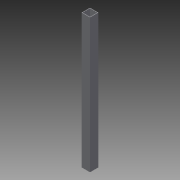
# Autodesk Inventor part: Part15-01
Saved by Autodesk Inventor 2013 (Build 170138000, 138)
## iProperties
Created: 2012-10-21
Part Number: Part15-01
Material: Generic
Document SubType Name: Modeling
Designer: Istvan
Density: 1 g/cm^3
Author: Istvan
Autodesk Inventor part; units mm, degrees
ref_plane "YZ Plane" through (0, 0, 0) normal (1, 0, 0) x (0, 1, 0)
ref_plane "XZ Plane" through (0, 0, 0) normal (0, 1, 0) x (-1, 0, 0)
ref_plane "XY Plane" through (0, 0, 0) normal (0, 0, 1) x (1, 0, 0)
sketch "Sketch1" plane through (0, 0, 0) normal (0, 1, 0) x (-1, 0, 0)
  line L0 (0, 0) -> (-38.1, 0)
  line L1 (-38.1, 0) -> (-38.1, -38.1)
  line L2 (-38.1, -38.1) -> (0, -38.1)
  line L3 (0, -38.1) -> (0, 0)
  line L4 (-35.7188, -35.7188) -> (-35.7188, -2.3812)
  line L5 (-35.7188, -2.3812) -> (-2.3813, -2.3813)
  line L6 (-2.3813, -2.3813) -> (-2.3812, -35.7188)
  line L7 (-2.3812, -35.7188) -> (-35.7188, -35.7188)
  dimension "d0" = 38.1
  dimension "d1" = 38.1
  dimension "d2" = 2.3813
  constraints: 16 end point, 4 parallel, 2 perpendicular, 1 horizontal, 3 other
  measures "d0" distance of L2.end L1.end
  measures "d1" distance of L1.end L0.end
  measures "d2" distance between parallel lines of L0 L5
extrude "Extrusion1" add sketch "Sketch1" along normal blind 609.6
equation "\"d0\" = d1"
body "Solid1"
